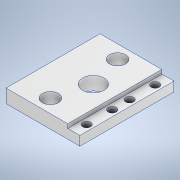
# Autodesk Inventor part: Piso, Vínculo Cabezal
Saved by Autodesk Inventor 2020 (Build 240168000, 168)
## iProperties
Created: 2020-05-11
Part Number: Piso, Vínculo Cabezal
Material: Aluminum 6061
Document SubType Name: Modeling
Designer: Dante
Density: 2.7 g/cm^3
Appearance: Aluminum - Flat
Mass: 85.1735 g
Surface Area: 108.497 cm^2
Volume: 31.5458 cm^3
Author: Dante
Autodesk Inventor part; units mm, degrees
ref_plane "YZ Plane" through (0, 0, 0) normal (1, 0, 0) x (0, 1, 0)
ref_plane "XZ Plane" through (0, 0, 0) normal (0, 1, 0) x (-1, 0, 0)
ref_plane "XY Plane" through (0, 0, 0) normal (0, 0, 1) x (1, 0, 0)
sketch "Sketch1" plane through (0, 0, 0) normal (0, 0, 1) x (1, 0, 0)
  line L0 (6.6074, 9.0814) -> (61.6074, 9.0814)
  line L1 (61.6074, 9.0814) -> (61.6074, 16.0814)
  line L2 (52.6074, 19.0814) -> (6.6074, 19.0814)
  line L3 (6.6074, 19.0814) -> (6.6074, 9.0814)
  line L4 (52.6074, 16.0814) -> (52.6074, 19.0814)
  line L5 (52.6074, 16.0814) -> (61.6074, 16.0814)
  dimension "d0" = 55
  dimension "d1" = 7
  dimension "d6" = 9
  dimension "d7" = 3
  constraints: 12 end point, 3 perpendicular, 2 horizontal, 1 vertical
  measures "d0" distance of L0.start L0.end
  measures "d1" distance of L0.end L1.end
  measures "d6" distance from line of L4.start L1
  measures "d7" distance of L2.start L4.start
extrude "Extrusion1" add sketch "Sketch1" along normal blind 70
sketch "Sketch2" plane through (6.6074, 19.0814, 0) normal (0, 1, 0) x (1, 0, 0)
  circle A0 centre (23, -10) radius 6
  circle A1 centre (23, -60) radius 6
  line L0 (46, -70) -> (0, -70) projected
  line L1 (55, 0) -> (55, -70) projected
  line L2 (46, 0) -> (0, 0) projected
  circle A2 centre (30, -35) radius 8
  line L3 (55, 0) -> (55, -70) projected
  circle A3 centre (50.5, -60.5) radius 3
  line L4 (46, 0) -> (46, -70) projected
  line L5 (55, -70) -> (46, -70) projected
  circle A4 centre (50.5, -41.5) radius 3
  circle A5 centre (50.5, -9.5) radius 3
  circle A6 centre (50.5, -28.5) radius 3
  line L6 (55, 0) -> (46, 0) projected
  point P0 (-6.6074, 0)
  dimension "d10" = 12
  dimension "d11" = 12
  dimension "d12" = 10
  dimension "d15" = 10
  dimension "d17" = 16
  dimension "d22" = 6
  dimension "d23" = 4.5
  dimension "d24" = 9.5
  dimension "d30" = 9.5
  dimension "d31" = 19
  dimension "d32" = 19
  dimension "d33" = 25
  dimension "d34" = 32
  dimension "d35" = 32
  dimension "d36" = 35
  dimension "d37" = 4.5
  dimension "d38" = 4.5
  dimension "d39" = 4.5
  constraints: 7 centre point
  measures "d10" diameter of A0
  measures "d11" diameter of A1
  measures "d12" distance from line of A1.centre L0
  measures "d15" distance from line of L2 A0.centre
  measures "d17" diameter of A2
  measures "d22" diameter of A3
  measures "d23" distance from line of A3.centre L4
  measures "d24" distance from line of L5 A3.centre
  measures "d30" distance from line of L6 A5.centre
  measures "d31" distance of A4.centre A3.centre
  measures "d32" distance of A5.centre A6.centre
  measures "d33" distance from line of L1 A2.centre
  measures "d34" distance from line of A1.centre L1
  measures "d35" distance from line of L3 A0.centre
  measures "d36" distance from line of L2 A2.centre
  measures "d37" distance from line of L4 A4.centre
  measures "d38" distance from line of A6.centre L4
  measures "d39" distance from line of A5.centre L4
extrude "Extrusion2" cut sketch "Sketch2" against normal blind 30 contours A0 | A1 | A2 | A3 | A4 | A5 | A6
body "Solid1"
